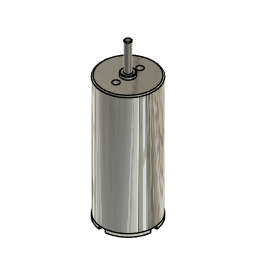
Coreless_Motor v2 (Autodesk Fusion 360 design; units mm, degrees)
Autodesk Fusion 360 part; units mm, degrees
sketch "Sketch1" plane through (0, 0, 0) normal (0, 0, 1) x (1, 0, 0)
  line L0 (196.5, 218.4641) -> (196.5, 218)
  line L1 (196.5, 218) -> (195.5, 218)
  line L2 (195.5, 218) -> (195.5, 218.4641)
  line L3 (191.7795, 214.7436) -> (192.2436, 214.7436)
  line L4 (192.2436, 214.7436) -> (192.2436, 213.7436)
  line L5 (192.2436, 213.7436) -> (191.7795, 213.7436)
  line L6 (195.5, 210.0231) -> (195.5, 210.4872)
  line L7 (195.5, 210.4872) -> (196.5, 210.4872)
  line L8 (196.5, 210.4872) -> (196.5, 210.0231)
  line L9 (200.2205, 213.7436) -> (199.7564, 213.7436)
  line L10 (199.7564, 213.7436) -> (199.7564, 214.7436)
  line L11 (199.7564, 214.7436) -> (200.2205, 214.7436)
  arc A0 (200.2205, 214.7436) -> (196.5, 218.4641) centre (196, 214.2436) ccw
  arc A1 (196.5, 210.0231) -> (200.2205, 213.7436) centre (196, 214.2436) ccw
  arc A2 (195.5, 218.4641) -> (191.7795, 214.7436) centre (196, 214.2436) ccw
  arc A3 (191.7795, 213.7436) -> (195.5, 210.0231) centre (196, 214.2436) ccw
  circle A4 centre (196, 216.2436) radius 0.5
  circle A5 centre (196, 212.2436) radius 0.5
  dimension "d1" = 8.5
  dimension "d6" = 0.5
  dimension "d8" = 360
  dimension "d9" = 0.4641
  dimension "d10" = 0.4641
  dimension "d14" = 1
  dimension "d15" = 1
  dimension "d16" = 2
  dimension "d17" = 2
  constraint vertical L0
  constraint horizontal L1
  constraint vertical L2
  constraint concentric A0 A2
  constraint concentric A1 A2
  constraint concentric A2 A3
  constraint collinear A0.centre A4.centre A5.centre
  measures "d1" diameter of A2
  measures "d6" distance of A0.centre L2
  measures "d9" distance of L3.start L3.end
  measures "d10" distance of L7.end L8.end
  measures "d14" diameter of A5
  measures "d15" diameter of A4
  measures "d16" distance of A0.centre A4.centre
  measures "d17" distance of A0.centre A5.centre
extrude "Extrude1" add sketch "Sketch1" along normal blind 0.5 makes body 1 in component "Motor Base Platic"
sketch "Sketch3" plane through (0, 0, 0.5) normal (0, 0, 1) x (-1, 0, 0)
  circle A0 centre (-196, -212.2436) radius 0.5
  circle A1 centre (-196, -216.2436) radius 0.5
  arc A2 (-191.7795, -213.7436) -> (-195.5, -210.0231) centre (-196, -214.2436) ccw
  line L0 (-195.5, -210.0231) -> (-195.5, -210.4872)
  line L1 (-195.5, -210.4872) -> (-196.5, -210.4872)
  line L2 (-196.5, -210.4872) -> (-196.5, -210.0231)
  arc A3 (-196.5, -210.0231) -> (-200.2205, -213.7436) centre (-196, -214.2436) ccw
  line L3 (-200.2205, -213.7436) -> (-199.7564, -213.7436)
  line L4 (-199.7564, -213.7436) -> (-199.7564, -214.7436)
  line L5 (-199.7564, -214.7436) -> (-200.2205, -214.7436)
  arc A4 (-200.2205, -214.7436) -> (-196.5, -218.4641) centre (-196, -214.2436) ccw
  line L6 (-196.5, -218.4641) -> (-196.5, -218)
  line L7 (-196.5, -218) -> (-195.5, -218)
  line L8 (-195.5, -218) -> (-195.5, -218.4641)
  arc A5 (-195.5, -218.4641) -> (-191.7795, -214.7436) centre (-196, -214.2436) ccw
  line L9 (-191.7795, -214.7436) -> (-192.2436, -214.7436)
  line L10 (-192.2436, -214.7436) -> (-192.2436, -213.7436)
  line L11 (-192.2436, -213.7436) -> (-191.7795, -213.7436)
  circle A6 centre (-196, -214.2436) radius 4.25
  dimension "d20" = 8.5
  constraint concentric A2 A6
  measures "d20" diameter of A6
extrude "Extrude1'" add sketch "Sketch3" along normal blind 19.5 separate body contours A0 | A1 | A2 L0 L1 L2 A3 L3 L4 L5 A4 L6 L7 L8 A5 L9 L10 L11 A6 | L9 L10 L11 A6 | L0 L1 L2 A6 | L3 L4 L5 A6 | L6 L7 L8 A6 makes body 2 in component "Motor Body"
sketch "Sketch4" plane through (0, 0, 20) normal (0, 0, 1) x (-1, 0, 0)
  circle A0 centre (-196, -214.2436) radius 4.25
  circle A1 centre (-196, -214.2436) radius 1
  circle A2 centre (-196, -214.2436) radius 0.55
  dimension "d23" = 2
  dimension "d24" = 1.1
  constraint concentric A0 A1
  constraint concentric A0 A2
  measures "d23" diameter of A1
  measures "d24" diameter of A2
extrude "Extrude2" add sketch "Sketch4" along normal blind 0.5 contours A1 bodies 2 in component "Motor Body"
fillet "Fillet1" radius 0.09 1 edges at (196.9323, 214.6052, 20.5) on bodies 2 in component "Motor Body"
sketch "Sketch5" plane through (0, 0, 20) normal (0, 0, 1) x (-1, 0, 0)
  circle A0 centre (-196, -214.2436) radius 0.55
  circle A1 centre (-196, -214.2436) radius 0.5
  dimension "d28" = 1
  constraint concentric A0 A1
  measures "d28" diameter of A1
extrude "Extrude1''" add sketch "Sketch5" along normal blind 5 separate body contours A1 makes body 3 in component "Motor Rotor"
sketch "Sketch6" plane through (0, 0, 20) normal (0, 0, 1) x (-1, 0, 0)
  circle A0 centre (-196, -214.2436) radius 4.25
  circle A1 centre (-196, -214.2436) radius 1
  circle A2 centre (-195.9641, -216.2436) radius 0.5
  circle A3 centre (-196.0359, -212.2436) radius 0.5
  point P0 (-196, -214.2436)
  dimension "d31" = 1
  dimension "d32" = 1
  dimension "d33" = 4
  dimension "d34" = 2
  constraint collinear A2.centre A3.centre P0
  measures "d31" diameter of A2
  measures "d32" diameter of A3
  measures "d33" vertical distance of A2.centre A3.centre
  measures "d34" vertical distance of A2.centre P0
extrude "Extrude3" cut sketch "Sketch6" against normal blind 5 contours A2 | A3 bodies 2 in component "Motor Body"
sketch "Sketch7" plane through (0, 0, 0.5) normal (0, 0, -1) x (1, 0, 0)
  circle A0 centre (196, -214.2436) radius 4.25
  circle A1 centre (196, -212.2436) radius 0.5
  circle A2 centre (196, -216.2436) radius 0.5
  point P0 (196, -212.2436)
  point P1 (196, -216.2436)
  dimension "d37" = 1
  dimension "d38" = 1
  dimension "d39" = 1
  constraint coincident P0 A1.centre
  constraint coincident P1 A2.centre
  measures "d37" diameter of A2
  measures "d38" diameter of A1
  measures "d39" diameter of A2
extrude "Extrude4" cut sketch "Sketch7" against normal blind 5 contours A1 | A2 bodies 2 in component "Motor Body"
fillet "Fillet1'" radius 0.1 1 edges at (196.4662, 214.4244, 25) on bodies 3 in component "Motor Rotor"
fillet "Fillet2" radius 0.2 1 edges at (199.9624, 215.7805, 20) on bodies 2 in component "Motor Body"
component "Motor Base Platic" placed x (1, 0, 0) y (0, -1, 0) z (0, 0, -1) at (-0.7905, 428.0822, 0.1145)
component "Motor Body" placed x (1, 0, 0) y (0, 1, 0) z (0, 0, 1) at (-0.7905, -0.4051, -0.3855)
component "Motor Rotor" placed x (1, 0, 0) y (0, 1, 0) z (0, 0, 1) at (-0.7905, -0.4051, -0.3855)
